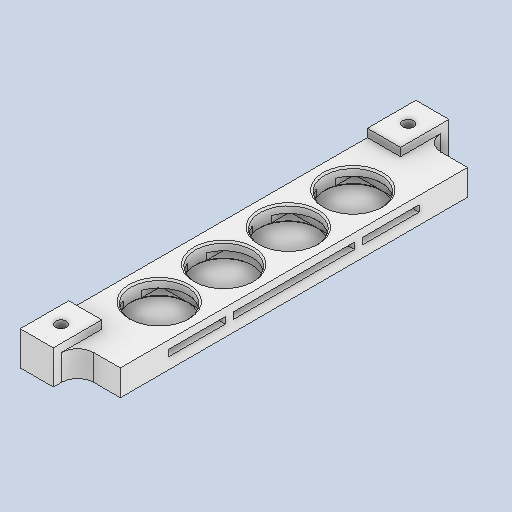
# Autodesk Inventor part: BatteryHolder
Saved by Autodesk Inventor 2023 (Build 270158000, 158)
## iProperties
Created: 2022-08-06
Part Number: BatteryHolder
Material: ABS Plastic
Document SubType Name: Modeling
Designer: Aditya Bansal
Density: 1.06 g/cm^3
Appearance: Smooth - White
Author: Aditya Bansal
Autodesk Inventor part; units mm, degrees
ref_plane "YZ Plane" through (0, 0, 0) normal (1, 0, 0) x (0, 1, 0)
ref_plane "XZ Plane" through (0, 0, 0) normal (0, 1, 0) x (-1, 0, 0)
ref_plane "XY Plane" through (0, 0, 0) normal (0, 0, 1) x (1, 0, 0)
sketch "Sketch1" plane through (0, 0, 0) normal (0, 1, 0) x (-1, 0, 0)
  line L0 (0, 0) -> (11.75, 0)
  line L1 (11.75, 0) -> (11.75, -107.5)
  line L2 (10.25, -107.5) -> (0, -107.5)
  line L3 (0, -107.5) -> (0, 0)
  circle A0 centre (11.75, -23.75) radius 8.75
  circle A1 centre (11.75, -43.75) radius 8.75
  circle A2 centre (11.75, -63.75) radius 8.75
  circle A3 centre (11.75, -83.75) radius 8.75
  line L4 (11.75, 0) -> (23.5, 0)
  line L5 (23.5, 0) -> (23.5, -107.5)
  line L6 (23.5, -107.5) -> (13.25, -107.5)
  line L7 (13.25, -107.5) -> (13.25, -92.3705)
  line L8 (13.25, -75.1295) -> (13.25, -72.3705)
  line L9 (13.25, -55.1295) -> (13.25, -52.3705)
  line L10 (13.25, -32.3705) -> (13.25, -35.1295)
  line L11 (13.25, -15.1295) -> (13.25, 0)
  line L12 (10.25, -52.3705) -> (10.25, -55.1295)
  line L13 (10.25, -107.5) -> (13.25, -107.5)
  line L14 (23.5, 0) -> (13.25, 0)
  line L15 (13.25, 0) -> (13.25, 7.5)
  line L16 (13.25, 7.5) -> (23.5, 7.5)
  line L17 (23.5, 7.5) -> (23.5, 0)
  line L18 (11.75, -107.5) -> (23.5, -107.5)
  line L19 (23.5, -107.5) -> (23.5, -115)
  line L20 (23.5, -115) -> (13.25, -115)
  line L21 (13.25, -115) -> (13.25, -107.5)
  point P0 (11.75, -92.5)
  point P1 (11.75, -75)
  point P2 (11.75, -72.5)
  point P3 (11.75, -55)
  point P4 (11.75, -52.5)
  point P5 (11.75, -35)
  point P6 (11.75, -32.5)
  point P7 (11.75, -15)
  dimension "d0" = 17.5
  dimension "d4" = 20
  dimension "d9" = 3
  dimension "d11" = 15
  dimension "d12" = 15
  dimension "d16" = 1.5
  dimension "d17" = 3
  dimension "d57" = 7.5
  constraints: 44 end point, 10 point on circle, 8 collinear, 8 point on line, 7 perpendicular, 6 parallel, 5 horizontal, 4 centre point, 2 vertical, 6 other
  measures "d0" diameter of A0
  measures "d4" distance of A0.centre A1.centre
  measures "d9" distance edge to line of A3 L3
  measures "d11" distance edge to line of A3 L2
  measures "d12" distance edge to line of A0 L0
  measures "d16" distance between parallel lines of L1 L7
  measures "d17" distance edge to line of A3 L5
  measures "d57" distance between parallel lines of L20 L6
extrude "Extrusion1" add sketch "Sketch1" along normal blind 5 contours L0 L1 A0 A1 L12 A2 A3 L13 L2 L3 | L4 L11 A0 L1 | L15 L16 L17 L4 | L4 L5 L6 L7 A3 L8 A2 L9 A1 L10 A0 L11 | A0 L10 A1 L1 | L1 A3 L7 L13 | L19 L20 L21 L6 | A1 L9 A2 L1 | L1 A2 L12 A1 | L1 A2 L8 A3
chamfer "Chamfer1" distance 0.5 angle 45 8 edges at (-10.25, 0, -92.3705) (-10.25, 0, -72.3705) (-10.25, 0, -52.3705) (-10.25, 0, -32.3705) (-10.25, 5, -32.3705) (-10.25, 5, -52.3705) (-10.25, 5, -72.3705) (-10.25, 5, -92.3705)
fillet "Fillet2" radius 5 2 edges at (-13.25, 2.5, -107.5) (-13.25, 2.5, 0)
sketch "Sketch5" plane through (0, 0, 0) normal (0, -1, 0) x (1, 0, 0)
  circle A0 centre (-11.75, -43.75) radius 9.25 construction
  circle A1 centre (-11.75, -83.75) radius 9.25 construction
  arc A2 (-8.25, -107.5) -> (-13.25, -112.5) centre (-8.25, -112.5) ccw projected
  line L0 (0, -107.5) -> (-8.25, -107.5) projected
  line L1 (0, 0) -> (0, -107.5) projected
  line L2 (-8.25, 0) -> (0, 0) projected
  arc A3 (-13.25, 5) -> (-8.25, 0) centre (-8.25, 5) ccw projected
  line L3 (-13.25, 7.5) -> (-13.25, 5) projected
  line L4 (-23.5, 7.5) -> (-13.25, 7.5) projected
  line L5 (-23.5, -115) -> (-23.5, 7.5) projected
  line L6 (-13.25, -115) -> (-23.5, -115) projected
  line L7 (-13.25, -112.5) -> (-13.25, -115) projected
  circle A4 centre (-11.75, -63.75) radius 9.25 construction
  circle A5 centre (-11.75, -23.75) radius 9.25 construction
extrude "Extrusion2" add sketch "Sketch5" along normal blind 3
sketch "Sketch6" plane through (0, 5, 0) normal (1, 0, 0) x (0, 0, -1)
  line L0 (52.5, -4.5) -> (35, -4.5) construction
  line L1 (35, -0.5) -> (52.5, -0.5) construction
  line L2 (72.5, -4.5) -> (55, -4.5) construction
  line L3 (55, -0.5) -> (72.5, -0.5) construction
  line L4 (52.5, -4.5) -> (35, -4.5) projected
  line L5 (72.5, -0.5) -> (72.5, -4.5) projected
  line L6 (35, -4.5) -> (72.5, -4.5)
  line L7 (72.5, -4.5) -> (72.5, -2.5)
  line L8 (72.5, -2.5) -> (35, -2.5)
  line L9 (35, -2.5) -> (35, -4.5)
  line L10 (15, -0.5) -> (32.5, -0.5) projected
  line L11 (75, -0.5) -> (92.5, -0.5) projected
  line L12 (32.5, -4.5) -> (15, -4.5) projected
  line L13 (92.5, -4.5) -> (75, -4.5) projected
  line L14 (32.5, -0.5) -> (32.5, -4.5) projected
  line L15 (15, -4.5) -> (32.5, -4.5)
  line L16 (32.5, -4.5) -> (32.5, -2.5)
  line L17 (32.5, -2.5) -> (15, -2.5)
  line L18 (15, -2.5) -> (15, -4.5)
  line L19 (92.5, -4.5) -> (75, -4.5)
  line L20 (75, -4.5) -> (75, -2.5)
  line L21 (75, -2.5) -> (92.5, -2.5)
  line L22 (92.5, -2.5) -> (92.5, -4.5)
  point P0 (0, -5)
  dimension "d61" = 2
  constraints: 24 end point, 6 parallel, 3 horizontal, 3 perpendicular, 2 midpoint, 1 point on line
  measures "d61" distance between parallel lines of L2 L8
extrude "Extrusion3" cut sketch "Sketch6" against normal blind 20
sketch "Sketch7" plane through (0, -3, 0) normal (0, -1, 0) x (1, 0, 0)
  circle A0 centre (-11.75, -23.75) radius 8.75 projected
  circle A1 centre (-11.75, -43.75) radius 8.75 projected
  circle A2 centre (-11.75, -63.75) radius 8.75 projected
  circle A3 centre (-11.75, -83.75) radius 8.75 projected
  line L0 (-16.75, -62.75) -> (-6.75, -62.75)
  line L1 (-6.75, -62.75) -> (-6.75, -64.75)
  line L2 (-6.75, -64.75) -> (-16.75, -64.75)
  line L3 (-16.75, -64.75) -> (-16.75, -62.75)
  line L4 (-16.75, -62.75) -> (-6.75, -64.75) construction
  line L5 (-6.75, -62.75) -> (-16.75, -64.75) construction
  line L6 (-10.75, -58.75) -> (-12.75, -58.75)
  line L7 (-12.75, -58.75) -> (-12.75, -68.75)
  line L8 (-12.75, -68.75) -> (-10.75, -68.75)
  line L9 (-10.75, -68.75) -> (-10.75, -58.75)
  line L10 (-10.75, -58.75) -> (-12.75, -68.75) construction
  line L11 (-12.75, -58.75) -> (-10.75, -68.75) construction
  line L12 (-10.75, -38.75) -> (-12.75, -38.75)
  line L13 (-12.75, -38.75) -> (-12.75, -48.75)
  line L14 (-12.75, -48.75) -> (-10.75, -48.75)
  line L15 (-10.75, -48.75) -> (-10.75, -38.75)
  line L16 (-10.75, -38.75) -> (-12.75, -48.75) construction
  line L17 (-12.75, -38.75) -> (-10.75, -48.75) construction
  line L18 (-16.75, -82.75) -> (-6.75, -82.75)
  line L19 (-6.75, -82.75) -> (-6.75, -84.75)
  line L20 (-6.75, -84.75) -> (-16.75, -84.75)
  line L21 (-16.75, -84.75) -> (-16.75, -82.75)
  line L22 (-16.75, -82.75) -> (-6.75, -84.75) construction
  line L23 (-6.75, -82.75) -> (-16.75, -84.75) construction
  line L24 (-10.75, -78.75) -> (-12.75, -78.75)
  line L25 (-12.75, -78.75) -> (-12.75, -88.75)
  line L26 (-12.75, -88.75) -> (-10.75, -88.75)
  line L27 (-10.75, -88.75) -> (-10.75, -78.75)
  line L28 (-10.75, -78.75) -> (-12.75, -88.75) construction
  line L29 (-12.75, -78.75) -> (-10.75, -88.75) construction
  line L30 (-10.75, -18.75) -> (-12.75, -18.75)
  line L31 (-12.75, -18.75) -> (-12.75, -28.75)
  line L32 (-12.75, -28.75) -> (-10.75, -28.75)
  line L33 (-10.75, -28.75) -> (-10.75, -18.75)
  line L34 (-10.75, -18.75) -> (-12.75, -28.75) construction
  line L35 (-12.75, -18.75) -> (-10.75, -28.75) construction
  point P0 (0, 0)
  point P1 (-10.75, -64.75)
  point P2 (-10.75, -62.75)
  point P3 (-12.75, -62.75)
  point P4 (-12.75, -64.75)
  point P5 (-12.75, -82.75)
  point P6 (-12.75, -84.75)
  point P7 (-10.75, -84.75)
  point P8 (-10.75, -82.75)
  dimension "d64" = 2
  dimension "d65" = 10
  dimension "d69" = 2
  dimension "d70" = 10
  constraints: 72 end point, 12 midpoint, 12 parallel, 7 equal length, 6 horizontal, 6 perpendicular, 2 coincident, 1 collinear
  measures "d64" distance of L7.end L8.end
  measures "d65" distance of L1.end L2.end
  measures "d69" distance of L26.start L26.end
  measures "d70" distance of L20.start L20.end
extrude "Extrusion4" cut sketch "Sketch7" against normal blind 0.5 contours L0 L7 L2 L3 | L7 L6 L9 L0 | L0 L9 L2 L7 | L0 L1 L2 L9 | L2 L9 L8 L7 | L15 L14 L13 L12 | L18 L25 L20 L21 | L25 L24 L27 L18 | L18 L27 L20 L25 | L18 L19 L20 L27 | L20 L27 L26 L25 | L33 L32 L31 L30
sketch "Sketch8" plane through (0, 5, 0) normal (0, 1, 0) x (1, 0, 0)
  line L0 (-23.5, -7.5) -> (-13.25, -7.5) projected
  line L1 (-23.5, -7.5) -> (-13.25, -7.5)
  line L2 (-13.25, -7.5) -> (-13.25, 7.5)
  line L3 (-13.25, 7.5) -> (-23.5, 7.5)
  line L4 (-23.5, 7.5) -> (-23.5, -7.5)
  line L5 (-13.25, -7.5) -> (-13.25, -5) projected
  line L6 (-23.5, 115) -> (-23.5, -7.5) projected
  line L7 (-23.5, 115) -> (-13.25, 115)
  line L8 (-13.25, 115) -> (-13.25, 100)
  line L9 (-13.25, 100) -> (-23.5, 100)
  line L10 (-23.5, 100) -> (-23.5, 115)
  line L11 (-13.25, 112.5) -> (-13.25, 115) projected
  point P0 (0, 0)
  dimension "d71" = 15
  dimension "d72" = 15
  constraints: 16 end point, 4 parallel, 2 collinear, 2 horizontal, 2 perpendicular
  measures "d71" distance of L3.end L0.start
  measures "d72" distance between parallel lines of L7 L9
extrude "Extrusion5" add sketch "Sketch8" along normal blind 2.5
sketch "Sketch4" plane through (0, -3, 0) normal (0, -1, 0) x (1, 0, 0)
  line L0 (-13.25, 7.5) -> (-23.5, 7.5) projected
  line L1 (-23.5, -115) -> (-13.25, -115) projected
  point P0 (0, 0)
  point P1 (-18.375, 0)
  point P2 (-18.375, -107.5)
  point P3 (-18.375, -115)
  point P4 (-18.375, 7.5)
  dimension "d53" = 7.5
  dimension "d68" = 7.5
  constraints: 3 midpoint, 2 vertical alignment
  measures "d53" distance of point (-18.375, -115) point (-18.375, -107.5)
  measures "d68" distance of point (-18.375, 0) point (-18.375, 7.5)
hole "Hole2" at (-18.375, -3, -107.5) at (-18.375, -3, 0) direction (0, 1, 0) diameter 3.4 end through all countersink diameter 6.3 countersink angle 90 clearance for "Flat Head Machine Screw" size "M3" standard "Ansi Metric M Profile"
equation "\"d12\" = d11"
body "Solid1"
